Autodesk Fusion 360 part; units mm, degrees
(part 4 of 4)
  line L1222 (-140.644, -87.9326) -> (-141.445, -87.9326)
  line L1223 (-141.445, -87.9326) -> (-141.445, -88.9331)
  line L1224 (-234.312, -31.7831) -> (-248.313, -31.7831)
  line L1225 (-248.313, -31.7831) -> (-248.313, -30.7827)
  line L1226 (-248.313, -30.7827) -> (-249.112, -30.7827)
  line L1227 (-249.112, -30.7827) -> (-249.112, -27.6848)
  line L1228 (-249.112, -27.6848) -> (-248.313, -27.6848)
  line L1229 (-248.313, -27.6848) -> (-248.313, -21.8833)
  line L1230 (-248.313, -21.8833) -> (-249.112, -21.8833)
  line L1231 (-249.112, -21.8833) -> (-249.112, -18.7827)
  line L1232 (-249.112, -18.7827) -> (-248.313, -18.7827)
  line L1233 (-248.313, -18.7827) -> (-248.313, -17.7836)
  line L1234 (-248.313, -17.7836) -> (-234.312, -17.7836)
  line L1235 (-234.312, -17.7836) -> (-234.312, -18.7827)
  line L1236 (-234.312, -18.7827) -> (-233.513, -18.7827)
  line L1237 (-233.513, -18.7827) -> (-233.513, -21.8833)
  line L1238 (-233.513, -21.8833) -> (-234.312, -21.8833)
  line L1239 (-234.312, -21.8833) -> (-234.312, -27.6848)
  line L1240 (-234.312, -27.6848) -> (-233.513, -27.6848)
  line L1241 (-233.513, -27.6848) -> (-233.513, -30.7827)
  line L1242 (-233.513, -30.7827) -> (-234.312, -30.7827)
  line L1243 (-234.312, -30.7827) -> (-234.312, -31.7831)
  line L1244 (-36.6697, -107.9831) -> (-50.669, -107.9831)
  line L1245 (-50.669, -107.9831) -> (-50.669, -106.9826)
  line L1246 (-50.669, -106.9826) -> (-51.4698, -106.9826)
  line L1247 (-51.4698, -106.9826) -> (-51.4698, -103.8834)
  line L1248 (-51.4698, -103.8834) -> (-50.669, -103.8834)
  line L1249 (-50.669, -103.8834) -> (-50.669, -98.0834)
  line L1250 (-50.669, -98.0834) -> (-51.4698, -98.0834)
  line L1251 (-51.4698, -98.0834) -> (-51.4698, -94.9828)
  line L1252 (-51.4698, -94.9828) -> (-50.669, -94.9828)
  line L1253 (-50.669, -94.9828) -> (-50.669, -93.9838)
  line L1254 (-50.669, -93.9838) -> (-36.6697, -93.9838)
  line L1255 (-36.6697, -93.9838) -> (-36.6697, -94.9828)
  line L1256 (-36.6697, -94.9828) -> (-35.869, -94.9828)
  line L1257 (-35.869, -94.9828) -> (-35.869, -98.0834)
  line L1258 (-35.869, -98.0834) -> (-36.6697, -98.0834)
  line L1259 (-36.6697, -98.0834) -> (-36.6697, -103.8834)
  line L1260 (-36.6697, -103.8834) -> (-35.869, -103.8834)
  line L1261 (-35.869, -103.8834) -> (-35.869, -106.9826)
  line L1262 (-35.869, -106.9826) -> (-36.6697, -106.9826)
  line L1263 (-36.6697, -106.9826) -> (-36.6697, -107.9831)
  line L1264 (-74.7697, -107.9831) -> (-88.769, -107.9831)
  line L1265 (-88.769, -107.9831) -> (-88.769, -106.9826)
  line L1266 (-88.769, -106.9826) -> (-89.5698, -106.9826)
  line L1267 (-89.5698, -106.9826) -> (-89.5698, -103.8834)
  line L1268 (-89.5698, -103.8834) -> (-88.769, -103.8834)
  line L1269 (-88.769, -103.8834) -> (-88.769, -98.0834)
  line L1270 (-88.769, -98.0834) -> (-89.5698, -98.0834)
  line L1271 (-89.5698, -98.0834) -> (-89.5698, -94.9828)
  line L1272 (-89.5698, -94.9828) -> (-88.769, -94.9828)
  line L1273 (-88.769, -94.9828) -> (-88.769, -93.9838)
  line L1274 (-88.769, -93.9838) -> (-74.7697, -93.9838)
  line L1275 (-74.7697, -93.9838) -> (-74.7697, -94.9828)
  line L1276 (-74.7697, -94.9828) -> (-73.9689, -94.9828)
  line L1277 (-73.9689, -94.9828) -> (-73.9689, -98.0834)
  line L1278 (-73.9689, -98.0834) -> (-74.7697, -98.0834)
  line L1279 (-74.7697, -98.0834) -> (-74.7697, -103.8834)
  line L1280 (-74.7697, -103.8834) -> (-73.9689, -103.8834)
  line L1281 (-73.9689, -103.8834) -> (-73.9689, -106.9826)
  line L1282 (-73.9689, -106.9826) -> (-74.7697, -106.9826)
  line L1283 (-74.7697, -106.9826) -> (-74.7697, -107.9831)
  line L1284 (-17.6197, -107.9831) -> (-31.6192, -107.9831)
  line L1285 (-31.6192, -107.9831) -> (-31.6192, -106.9826)
  line L1286 (-31.6192, -106.9826) -> (-32.4198, -106.9826)
  line L1287 (-32.4198, -106.9826) -> (-32.4198, -103.8834)
  line L1288 (-32.4198, -103.8834) -> (-31.6192, -103.8834)
  line L1289 (-31.6192, -103.8834) -> (-31.6192, -98.0834)
  line L1290 (-31.6192, -98.0834) -> (-32.4198, -98.0834)
  line L1291 (-32.4198, -98.0834) -> (-32.4198, -94.9828)
  line L1292 (-32.4198, -94.9828) -> (-31.6192, -94.9828)
  line L1293 (-31.6192, -94.9828) -> (-31.6192, -93.9838)
  line L1294 (-31.6192, -93.9838) -> (-17.6197, -93.9838)
  line L1295 (-17.6197, -93.9838) -> (-17.6197, -94.9828)
  line L1296 (-17.6197, -94.9828) -> (-16.819, -94.9828)
  line L1297 (-16.819, -94.9828) -> (-16.819, -98.0834)
  line L1298 (-16.819, -98.0834) -> (-17.6197, -98.0834)
  line L1299 (-17.6197, -98.0834) -> (-17.6197, -103.8834)
  line L1300 (-17.6197, -103.8834) -> (-16.819, -103.8834)
  line L1301 (-16.819, -103.8834) -> (-16.819, -106.9826)
  line L1302 (-16.819, -106.9826) -> (-17.6197, -106.9826)
  line L1303 (-17.6197, -106.9826) -> (-17.6197, -107.9831)
  line L1304 (-231.932, -50.833) -> (-245.932, -50.833)
  line L1305 (-245.932, -50.833) -> (-245.932, -49.8327)
  line L1306 (-245.932, -49.8327) -> (-246.731, -49.8327)
  line L1307 (-246.731, -49.8327) -> (-246.731, -46.7348)
  line L1308 (-246.731, -46.7348) -> (-245.932, -46.7348)
  line L1309 (-245.932, -46.7348) -> (-245.932, -40.9333)
  line L1310 (-245.932, -40.9333) -> (-246.731, -40.9333)
  line L1311 (-246.731, -40.9333) -> (-246.731, -37.8327)
  line L1312 (-246.731, -37.8327) -> (-245.932, -37.8327)
  line L1313 (-245.932, -37.8327) -> (-245.932, -36.8336)
  line L1314 (-245.932, -36.8336) -> (-231.932, -36.8336)
  line L1315 (-231.932, -36.8336) -> (-231.932, -37.8327)
  line L1316 (-231.932, -37.8327) -> (-231.131, -37.8327)
  line L1317 (-231.131, -37.8327) -> (-231.131, -40.9333)
  line L1318 (-231.131, -40.9333) -> (-231.932, -40.9333)
  line L1319 (-231.932, -40.9333) -> (-231.932, -46.7348)
  line L1320 (-231.932, -46.7348) -> (-231.131, -46.7348)
  line L1321 (-231.131, -46.7348) -> (-231.131, -49.8327)
  line L1322 (-231.131, -49.8327) -> (-231.932, -49.8327)
  line L1323 (-231.932, -49.8327) -> (-231.932, -50.833)
  line L1324 (-29.5259, -50.833) -> (-43.5254, -50.833)
  line L1325 (-43.5254, -50.833) -> (-43.5254, -49.8327)
  line L1326 (-43.5254, -49.8327) -> (-44.326, -49.8327)
  line L1327 (-44.326, -49.8327) -> (-44.326, -46.7348)
  line L1328 (-44.326, -46.7348) -> (-43.5254, -46.7348)
  line L1329 (-43.5254, -46.7348) -> (-43.5254, -46.1326)
  line L1330 (-43.5254, -46.1326) -> (-45.0509, -46.1326)
  line L1331 (-45.0509, -46.1326) -> (-45.0509, -49.3628)
  line L1332 (-45.0509, -49.3628) -> (-46.7748, -49.3628)
  line L1333 (-46.7748, -49.3628) -> (-46.7748, -50.2848)
  line L1334 (-46.7748, -50.2848) -> (-50.0752, -50.2848)
  line L1335 (-50.0752, -50.2848) -> (-50.0752, -49.3628)
  line L1336 (-50.0752, -49.3628) -> (-51.8004, -49.3628)
  line L1337 (-51.8004, -49.3628) -> (-51.8004, -46.1326)
  line L1338 (-51.8004, -46.1326) -> (-52.6259, -46.1326)
  line L1339 (-52.6259, -46.1326) -> (-52.6259, -43.3338)
  line L1340 (-52.6259, -43.3338) -> (-51.8004, -43.3338)
  line L1341 (-51.8004, -43.3338) -> (-51.8004, -37.0638)
  line L1342 (-51.8004, -37.0638) -> (-50.0752, -37.0638)
  line L1343 (-50.0752, -37.0638) -> (-50.0752, -36.0826)
  line L1344 (-50.0752, -36.0826) -> (-46.7748, -36.0826)
  line L1345 (-46.7748, -36.0826) -> (-46.7748, -37.0638)
  line L1346 (-46.7748, -37.0638) -> (-45.0509, -37.0638)
  line L1347 (-45.0509, -37.0638) -> (-45.0509, -41.5327)
  line L1348 (-45.0509, -41.5327) -> (-43.5254, -41.5327)
  line L1349 (-43.5254, -41.5327) -> (-43.5254, -40.9333)
  line L1350 (-43.5254, -40.9333) -> (-44.326, -40.9333)
  line L1351 (-44.326, -40.9333) -> (-44.326, -37.8327)
  line L1352 (-44.326, -37.8327) -> (-43.5254, -37.8327)
  line L1353 (-43.5254, -37.8327) -> (-43.5254, -36.8336)
  line L1354 (-43.5254, -36.8336) -> (-29.5259, -36.8336)
  line L1355 (-29.5259, -36.8336) -> (-29.5259, -37.8327)
  line L1356 (-29.5259, -37.8327) -> (-28.7253, -37.8327)
  line L1357 (-28.7253, -37.8327) -> (-28.7253, -40.9333)
  line L1358 (-28.7253, -40.9333) -> (-29.5259, -40.9333)
  line L1359 (-29.5259, -40.9333) -> (-29.5259, -41.5327)
  line L1360 (-29.5259, -41.5327) -> (-28.0004, -41.5327)
  line L1361 (-28.0004, -41.5327) -> (-28.0004, -37.0638)
  line L1362 (-28.0004, -37.0638) -> (-26.2751, -37.0638)
  line L1363 (-26.2751, -37.0638) -> (-26.2751, -36.0826)
  line L1364 (-26.2751, -36.0826) -> (-22.9761, -36.0826)
  line L1365 (-22.9761, -36.0826) -> (-22.9761, -37.0638)
  line L1366 (-22.9761, -37.0638) -> (-21.2508, -37.0638)
  line L1367 (-21.2508, -37.0638) -> (-21.2508, -43.3338)
  line L1368 (-21.2508, -43.3338) -> (-20.4253, -43.3338)
  line L1369 (-20.4253, -43.3338) -> (-20.4253, -46.1326)
  line L1370 (-20.4253, -46.1326) -> (-21.2508, -46.1326)
  line L1371 (-21.2508, -46.1326) -> (-21.2508, -49.3628)
  line L1372 (-21.2508, -49.3628) -> (-22.9761, -49.3628)
  line L1373 (-22.9761, -49.3628) -> (-22.9761, -50.2848)
  line L1374 (-22.9761, -50.2848) -> (-26.2751, -50.2848)
  line L1375 (-26.2751, -50.2848) -> (-26.2751, -49.3628)
  line L1376 (-26.2751, -49.3628) -> (-28.0004, -49.3628)
  line L1377 (-28.0004, -49.3628) -> (-28.0004, -46.1326)
  line L1378 (-28.0004, -46.1326) -> (-29.5259, -46.1326)
  line L1379 (-29.5259, -46.1326) -> (-29.5259, -46.7348)
  line L1380 (-29.5259, -46.7348) -> (-28.7253, -46.7348)
  line L1381 (-28.7253, -46.7348) -> (-28.7253, -49.8327)
  line L1382 (-28.7253, -49.8327) -> (-29.5259, -49.8327)
  line L1383 (-29.5259, -49.8327) -> (-29.5259, -50.833)
  line L1384 (-203.357, -69.8831) -> (-217.357, -69.8831)
  line L1385 (-217.357, -69.8831) -> (-217.357, -68.8826)
  line L1386 (-217.357, -68.8826) -> (-218.156, -68.8826)
  line L1387 (-218.156, -68.8826) -> (-218.156, -65.7834)
  line L1388 (-218.156, -65.7834) -> (-217.357, -65.7834)
  line L1389 (-217.357, -65.7834) -> (-217.357, -59.9834)
  line L1390 (-217.357, -59.9834) -> (-218.156, -59.9834)
  line L1391 (-218.156, -59.9834) -> (-218.156, -56.8828)
  line L1392 (-218.156, -56.8828) -> (-217.357, -56.8828)
  line L1393 (-217.357, -56.8828) -> (-217.357, -55.8838)
  line L1394 (-217.357, -55.8838) -> (-203.357, -55.8838)
  line L1395 (-203.357, -55.8838) -> (-203.357, -56.8828)
  line L1396 (-203.357, -56.8828) -> (-202.556, -56.8828)
  line L1397 (-202.556, -56.8828) -> (-202.556, -59.9834)
  line L1398 (-202.556, -59.9834) -> (-203.357, -59.9834)
  line L1399 (-203.357, -59.9834) -> (-203.357, -65.7834)
  line L1400 (-203.357, -65.7834) -> (-202.556, -65.7834)
  line L1401 (-202.556, -65.7834) -> (-202.556, -68.8826)
  line L1402 (-202.556, -68.8826) -> (-203.357, -68.8826)
  line L1403 (-203.357, -68.8826) -> (-203.357, -69.8831)
  line L1404 (-279.557, -88.9331) -> (-293.557, -88.9331)
  line L1405 (-293.557, -88.9331) -> (-293.557, -87.9326)
  line L1406 (-293.557, -87.9326) -> (-294.356, -87.9326)
  line L1407 (-294.356, -87.9326) -> (-294.356, -84.8334)
  line L1408 (-294.356, -84.8334) -> (-293.557, -84.8334)
  line L1409 (-293.557, -84.8334) -> (-293.557, -79.0334)
  line L1410 (-293.557, -79.0334) -> (-294.356, -79.0334)
  line L1411 (-294.356, -79.0334) -> (-294.356, -75.9328)
  line L1412 (-294.356, -75.9328) -> (-293.557, -75.9328)
  line L1413 (-293.557, -75.9328) -> (-293.557, -74.9338)
  line L1414 (-293.557, -74.9338) -> (-279.557, -74.9338)
  line L1415 (-279.557, -74.9338) -> (-279.557, -75.9328)
  line L1416 (-279.557, -75.9328) -> (-278.756, -75.9328)
  line L1417 (-278.756, -75.9328) -> (-278.756, -79.0334)
  line L1418 (-278.756, -79.0334) -> (-279.557, -79.0334)
  line L1419 (-279.557, -79.0334) -> (-279.557, -84.8334)
  line L1420 (-279.557, -84.8334) -> (-278.756, -84.8334)
  line L1421 (-278.756, -84.8334) -> (-278.756, -87.9326)
  line L1422 (-278.756, -87.9326) -> (-279.557, -87.9326)
  line L1423 (-279.557, -87.9326) -> (-279.557, -88.9331)
  line L1424 (-83.5812, -113.8054) -> (-244.3297, -113.8054) construction
  line L1425 (-244.3297, -113.8054) -> (-244.3297, -140.9865) construction
  line L1426 (-244.3297, -140.9865) -> (-83.5812, -140.9865) construction
  line L1427 (-83.5812, -140.9865) -> (-83.5812, -113.8054) construction
  dimension "d49" = 20
  text T0 "MechaCore" font "Arial" height 20 align left top in box 160.7485 x 27.1811 at (-83.5812, -113.8054) x (-1, 0) y (0, -1) spacing 1 kerned
extrude "Extrude12" cut sketch "Sketch4" against normal blind 0.5 text T0 bodies 2
extrude "Extrude13" cut 1 faces at (0.6667, 7.0667, -128.8) along direction (0, -0.67828, -0.734803) blind 1.5 on bodies 1 bodies 1
extrude "Extrude14" cut 1 faces at (0.6667, 6.2, -126.1) along direction (0, -1, 0) blind 1.5 on bodies 1 bodies 1
extrude "Extrude15" cut 1 faces at (0.6667, 5.7, -128) along direction (0, 0, -1) blind 1.5 on bodies 1 bodies 1
extrude "Extrude16" cut 1 faces at (0.6667, 8.6333, -129.2) along direction (0, 0, -1) blind 1.5 on bodies 1 bodies 1
extrude "Extrude17" cut 1 faces at (0.6667, 7.5, -129.7) along direction (0, -1, 0) blind 2.8 on bodies 1 bodies 1
extrude "Extrude18" cut 1 faces at (0.6667, 5.7, -122.3) along direction (0, 0, 1) blind 1.5 on bodies 1 bodies 1
extrude "Extrude19" cut 1 faces at (0.6667, 6.2, -121.8) along direction (0, 1, 0) blind 3 on bodies 1 bodies 1
equation "d50 = 'MechaCore'"
